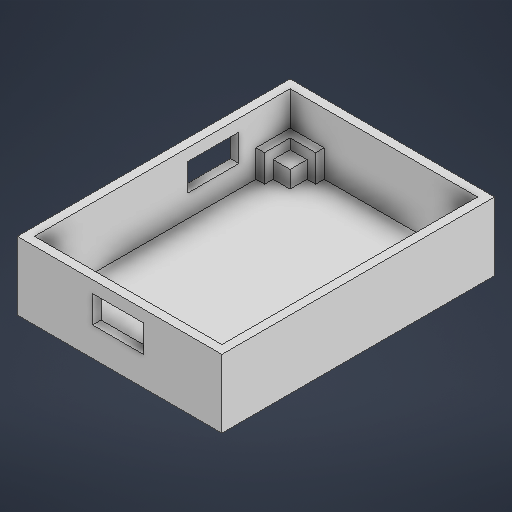
# Autodesk Inventor part: Caixa
Saved by Autodesk Inventor 2025 (Build 290162010, 162A)
## iProperties
Created: 2024-07-28
Part Number: Caixa
Material: Generic
Document SubType Name: Modeling
Designer: GabrielDBN
Density: 1 g/cm^3
Appearance: Default
Author: GabrielDBN
Autodesk Inventor part; units mm, degrees
ref_plane "YZ Plane" through (0, 0, 0) normal (1, 0, 0) x (0, 1, 0)
ref_plane "XZ Plane" through (0, 0, 0) normal (0, 1, 0) x (-1, 0, 0)
ref_plane "XY Plane" through (0, 0, 0) normal (0, 0, 1) x (1, 0, 0)
sketch "Sketch1" plane through (0, 0, 0) normal (0, 1, 0) x (-1, 0, 0)
  line L0 (27.0344, 35.8723) -> (-27.9656, 35.8723)
  line L1 (27.0344, 35.8723) -> (27.0344, -39.1277)
  line L2 (27.0344, -39.1277) -> (-27.9656, -39.1277)
  line L3 (-27.9656, -39.1277) -> (-27.9656, 35.8723)
  line L4 (24.5344, 33.3723) -> (22.0344, 33.3723)
  line L5 (-25.4656, -36.6277) -> (-22.9656, -36.6277)
  line L6 (-25.4656, -36.6277) -> (-25.4656, -34.1277)
  line L7 (24.5344, -36.6277) -> (22.0344, -36.6277)
  line L8 (24.5344, -36.6277) -> (24.5344, -34.1277)
  line L9 (24.5344, 30.8723) -> (24.5344, 33.3723)
  line L10 (22.0344, 33.3723) -> (19.5344, 33.3723)
  line L11 (24.5344, 30.8723) -> (24.5344, 28.3723)
  line L12 (24.5344, 28.3723) -> (19.5344, 28.3723)
  line L13 (19.5344, 28.3723) -> (19.5344, 33.3723)
  line L14 (-20.4656, 33.3723) -> (-20.4656, 28.3723)
  line L15 (-20.4656, 28.3723) -> (-25.4656, 28.3723)
  line L16 (22.0344, -36.6277) -> (19.5344, -36.6277)
  line L17 (19.5344, -36.6277) -> (19.5344, -31.6277)
  line L18 (19.5344, -31.6277) -> (24.5344, -31.6277)
  line L19 (24.5344, -31.6277) -> (24.5344, -34.1277)
  line L20 (-22.9656, -36.6277) -> (-20.4656, -36.6277)
  line L21 (-20.4656, -36.6277) -> (-20.4656, -31.6277)
  line L22 (-20.4656, -31.6277) -> (-25.4656, -31.6277)
  line L23 (-25.4656, -31.6277) -> (-25.4656, -34.1277)
  line L24 (-30.4656, -41.6277) -> (-30.4656, 38.3723)
  line L25 (-30.4656, -41.6277) -> (29.5344, -41.6277)
  line L26 (29.5344, -41.6277) -> (29.5344, 38.3723)
  line L27 (29.5344, 38.3723) -> (-30.4656, 38.3723)
  line L28 (-20.4656, 33.3723) -> (-25.4656, 33.3723)
  line L29 (-25.4656, 33.3723) -> (-25.4656, 28.3723)
  point P0 (0, 0)
  dimension "d1" = 55
  dimension "d2" = 75
  dimension "d34" = 80
  dimension "d35" = 60
  dimension "d36" = 5
  constraints: 60 end point, 14 perpendicular, 7 horizontal, 5 vertical, 1 collinear
  measures "d1" distance of L0.start L0.end
  measures "d2" distance of L0.start L1.end
  measures "d34" distance of L25.end L26.end
  measures "d35" distance of L26.end L24.end
  measures "d36" distance of L28.end L15.end
extrude "Extrusion1" add sketch "Sketch1" along normal blind 2 contours L1 L2 L3 L0
extrude "Extrusion2" add sketch "Sketch1" along normal blind 7 contours L9 L11 L12 L13 L10 L4 | L6 L23 L22 L21 L20 L5 | L7 L16 L17 L18 L19 L8 | L14 L15 L29 L28
extrude "Extrusion3" add sketch "Sketch1" along normal blind 20 contours L24 L27 L26 L25
sketch "Sketch2" plane through (-29.5344, 0, 38.3723) normal (0, 0, 1) x (1, 0, 0)
  line L0 (55, 7) -> (50, 7) projected
  line L1 (52.5, 7) -> (52.5, 8.5)
  line L2 (10, 7) -> (5, 7) projected
  line L3 (5, 7) -> (5, 8.5)
  line L4 (29.5344, 8.5) -> (37.0344, 8.5)
  line L5 (37.0344, 8.5) -> (37.0344, 16.5)
  line L6 (37.0344, 16.5) -> (22.0344, 16.5)
  line L7 (22.0344, 16.5) -> (22.0344, 8.5)
  line L8 (22.0344, 8.5) -> (29.5344, 8.5)
  point P0 (29.5344, 0)
  dimension "d43" = 1.5
  constraints: 14 end point, 4 perpendicular, 2 vertical, 1 horizontal, 1 midpoint, 1 point on line
  measures "d43" distance of L1.start L1.end
extrude "Extrusion4" cut sketch "Sketch2" against normal blind 10
sketch "Sketch3" plane through (0, 2, 0) normal (0, 1, 0) x (1, 0, 0)
  line L0 (-24.5344, 36.6277) -> (-19.5344, 36.6277) projected
  line L1 (-17.0344, 36.6277) -> (-17.0344, 39.1277)
  line L2 (27.9656, 39.1277) -> (-27.0344, 39.1277) projected
  line L3 (-17.0344, 39.1277) -> (-27.0344, 39.1277)
  line L4 (-24.5344, 29.1277) -> (-27.0344, 29.1277)
  line L5 (-27.0344, 39.1277) -> (-27.0344, -35.8723) projected
  line L6 (-27.0344, 29.1277) -> (-27.0344, 39.1277)
  line L7 (-24.5344, 36.6277) -> (-24.5344, 31.6277) projected
  line L8 (-17.0344, 36.6277) -> (-24.5344, 36.6277)
  line L9 (-24.5344, 36.6277) -> (-24.5344, 29.1277)
  line L10 (27.9656, 39.1277) -> (17.9656, 39.1277)
  line L11 (27.9656, 39.1277) -> (27.9656, 29.1277)
  line L12 (27.9656, -35.8723) -> (27.9656, 39.1277) projected
  line L13 (17.9656, 39.1277) -> (17.9656, 36.6277)
  line L14 (25.4656, 36.6277) -> (20.4656, 36.6277) projected
  line L15 (17.9656, 36.6277) -> (25.4656, 36.6277)
  line L16 (25.4656, 36.6277) -> (25.4656, 29.1277)
  line L17 (25.4656, 29.1277) -> (27.9656, 29.1277)
  line L18 (-27.0344, -35.8723) -> (27.9656, -35.8723) projected
  line L19 (27.9656, -35.8723) -> (27.9656, -25.8723)
  line L20 (27.9656, -35.8723) -> (17.9656, -35.8723)
  line L21 (20.4656, -33.3723) -> (25.4656, -33.3723) projected
  line L22 (27.9656, -25.8723) -> (25.4656, -25.8723)
  line L23 (25.4656, -28.3723) -> (25.4656, -33.3723) projected
  line L24 (25.4656, -25.8723) -> (25.4656, -33.3723)
  line L25 (17.9656, -35.8723) -> (17.9656, -33.3723)
  line L26 (25.4656, -33.3723) -> (20.4656, -33.3723) projected
  line L27 (17.9656, -33.3723) -> (25.4656, -33.3723)
  line L28 (-27.0344, -35.8723) -> (-27.0344, -25.8723)
  line L29 (-27.0344, -35.8723) -> (-17.0344, -35.8723)
  line L30 (-17.0344, -35.8723) -> (-17.0344, -33.3723)
  line L31 (-17.0344, -33.3723) -> (-24.5344, -33.3723)
  line L32 (-24.5344, -33.3723) -> (-24.5344, -25.8723)
  line L33 (-24.5344, -25.8723) -> (-27.0344, -25.8723)
  point P0 (0, 0)
  constraints: 48 end point, 8 point on line, 7 perpendicular, 4 collinear, 3 vertical, 2 horizontal
extrude "Extrusion5" add sketch "Sketch3" along normal blind 8 contours L7 L9 L4 L5 L2 L1 L8 L0
extrude "Extrusion6" add sketch "Sketch3" along normal blind 8 contours L2 L11 L17 L16 L14 L15 L13
extrude "Extrusion7" add sketch "Sketch3" along normal blind 8 contours L12 L18 L25 L27 L21 L23 L24 L22
extrude "Extrusion8" add sketch "Sketch3" along normal blind 8 contours L33 L32 L31 L30 L18 L5
sketch "Sketch4" plane through (-29.5344, 0, -41.6277) normal (-1, 0, 0) x (0, 0, 1)
  line L0 (0, 0) -> (0, 20) projected
  line L1 (17.5, 8.5) -> (17.5, 16.5)
  line L2 (17.5, 16.5) -> (32.5, 16.5)
  line L3 (32.5, 16.5) -> (32.5, 8.5)
  line L4 (17.5, 8.5) -> (32.5, 8.5)
  point P0 (41.6277, 0)
  constraints: 8 end point, 2 horizontal, 1 vertical
extrude "Extrusion9" cut sketch "Sketch4" against normal blind 5
body "Solid1"
